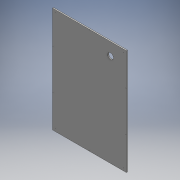
# Autodesk Inventor part: Plateau
Saved by Autodesk Inventor 2016 SP1 (Build 200210100, 210)
## iProperties
Created: 2017-04-24
Part Number: Plateau
Material: Bois (bouleau)
Document SubType Name: Modeling
Designer: dimercur
Density: 0.55 g/cm^3
Appearance: Par défaut
Author: dimercur
Autodesk Inventor part; units mm, degrees
ref_plane "YZ Plane" through (0, 0, 0) normal (1, 0, 0) x (0, 1, 0)
ref_plane "XZ Plane" through (0, 0, 0) normal (0, 1, 0) x (-1, 0, 0)
ref_plane "XY Plane" through (0, 0, 0) normal (0, 0, 1) x (1, 0, 0)
sketch "Esquisse1" plane through (0, 0, 0) normal (0, 1, 0) x (-1, 0, 0)
  line L0 (350, 500) -> (-350, 500)
  line L1 (-350, 500) -> (-350, -500)
  line L2 (-350, -500) -> (350, -500)
  line L3 (350, -500) -> (350, 500)
  point P0 (0, 0)
  dimension "d0" = 1000
  dimension "d1" = 700
  dimension "d2" = 350
  dimension "d3" = 500
  constraints: 8 end point, 2 parallel, 1 horizontal, 1 perpendicular
  measures "d0" distance of L2.end L0.start
  measures "d1" distance of L0.start L0.end
  measures "d2" horizontal distance of point (0, 0) L0.start
  measures "d3" vertical distance of point (0, 0) L0.start
extrude "Extrusion1" add sketch "Esquisse1" along normal blind 10
sketch "Esquisse2" plane through (0, 10, 0) normal (0, 1, 0) x (1, 0, 0)
  point P0 (0, 0)
sketch "Esquisse3" plane through (0, 10, 0) normal (0, 1, 0) x (1, 0, 0)
  point P0 (0, 0)
sketch "Esquisse4" plane through (0, 10, 0) normal (0, 1, 0) x (1, 0, 0)
  circle A0 centre (200, -380) radius 27.5
  line L0 (-350, -500) -> (350, -500) projected
  line L1 (350, -500) -> (350, 500) projected
  point P0 (0, 0)
  dimension "d6" = 55
  dimension "d7" = 120
  dimension "d8" = 150
  constraints: 1 centre point
  measures "d6" diameter of A0
  measures "d7" distance from line of L0 A0.centre
  measures "d8" distance from line of L1 A0.centre
extrude "Extrusion2" cut sketch "Esquisse4" against normal through all
sketch "Esquisse5" plane through (0, 10, 0) normal (0, 1, 0) x (1, 0, 0)
  circle A0 centre (-325, -475) radius 1.5
  circle A1 centre (325, -475) radius 1.5
  circle A2 centre (325, 475) radius 1.5
  circle A3 centre (-325, 475) radius 1.5
  line L0 (350, 500) -> (-350, 500) projected
  line L1 (350, -500) -> (350, 500) projected
  line L2 (-350, 500) -> (-350, -500) projected
  line L3 (-350, -500) -> (350, -500) projected
  circle A4 centre (-345, -190) radius 1.5
  circle A5 centre (-345, 190) radius 1.5
  circle A6 centre (0, -495) radius 1.5
  circle A7 centre (0, 495) radius 1.5
  circle A8 centre (345, -190) radius 1.5
  circle A9 centre (345, 190) radius 1.5
  point P0 (0, 0)
  dimension "d11" = 3
  dimension "d12" = 3
  dimension "d13" = 3
  dimension "d14" = 3
  dimension "d15" = 25
  dimension "d16" = 25
  dimension "d17" = 25
  dimension "d18" = 25
  dimension "d19" = 25
  dimension "d20" = 25
  dimension "d21" = 25
  dimension "d22" = 25
  dimension "d23" = 3
  dimension "d24" = 3
  dimension "d25" = 3
  dimension "d26" = 3
  dimension "d27" = 3
  dimension "d28" = 3
  dimension "d29" = 5
  dimension "d30" = 5
  dimension "d31" = 5
  dimension "d32" = 5
  dimension "d33" = 5
  dimension "d34" = 5
  dimension "d35" = 350
  dimension "d36" = 350
  dimension "d37" = 190
  dimension "d38" = 190
  dimension "d39" = 190
  dimension "d40" = 190
  constraints: 10 centre point
  measures "d11" diameter of A3
  measures "d12" diameter of A0
  measures "d13" diameter of A1
  measures "d14" diameter of A2
  measures "d15" distance from line of L0 A2.centre
  measures "d16" distance from line of L1 A2.centre
  measures "d17" distance from line of L0 A3.centre
  measures "d18" distance from line of L2 A3.centre
  measures "d19" distance from line of L3 A0.centre
  measures "d20" distance from line of L2 A0.centre
  measures "d21" distance from line of L1 A1.centre
  measures "d22" distance from line of L3 A1.centre
  measures "d23" diameter of A4
  measures "d24" diameter of A5
  measures "d25" diameter of A6
  measures "d26" diameter of A8
  measures "d27" diameter of A9
  measures "d28" diameter of A7
  measures "d29" distance from line of L2 A4.centre
  measures "d30" distance from line of L2 A5.centre
  measures "d31" distance from line of L3 A6.centre
  measures "d32" distance from line of L0 A7.centre
  measures "d33" distance from line of L1 A9.centre
  measures "d34" distance from line of L1 A8.centre
  measures "d35" distance from line of L2 A6.centre
  measures "d36" distance from line of L2 A7.centre
  measures "d37" vertical distance of point (0, 0) A8.centre
  measures "d38" vertical distance of point (0, 0) A9.centre
  measures "d39" vertical distance of point (0, 0) A4.centre
  measures "d40" vertical distance of A5.centre point (0, 0)
extrude "Extrusion3" cut sketch "Esquisse5" against normal through all contours A0 | A1 | A2 | A3 | A4 | A5 | A6 | A7 | A8 | A9
equation "\"d0\" = Longueur_Plateau"
equation "\"d1\" = Largeur_Plateau"
equation "\"d2\" = 0.5 * d1"
equation "\"d3\" = 0.5 * d0"
equation "\"d12\" = d11"
equation "\"d13\" = d11"
equation "\"d14\" = d11"
equation "\"d16\" = d15"
equation "\"d17\" = d15"
equation "\"d18\" = d15"
equation "\"d19\" = d15"
equation "\"d20\" = d15"
equation "\"d21\" = d15"
equation "\"d22\" = d15"
equation "\"d24\" = d23"
equation "\"d25\" = d23"
equation "\"d26\" = d23"
equation "\"d27\" = d23"
equation "\"d28\" = d23"
equation "\"d30\" = d29"
equation "\"d31\" = d29"
equation "\"d32\" = d29"
equation "\"d33\" = d29"
equation "\"d34\" = d29"
equation "\"d38\" = d37"
equation "\"d39\" = d37"
equation "\"d40\" = d37"
equation "\"Longueur_Plateau\" = 1000"
equation "\"Largeur_Plateau\" = 700"
